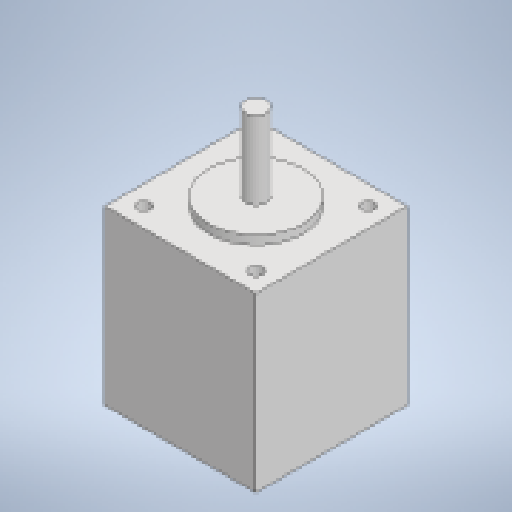
# Autodesk Inventor part: 35x40 stepper
Saved by Autodesk Inventor 2025 (Build 290162000, 162)
## iProperties
Created: 2025-09-03
Part Number: 35x40 stepper
Material: 一般
Document SubType Name: Modeling
Designer: gavin
Density: 1 g/cm^3
Appearance: 預設
Author: gavin
Autodesk Inventor part; units mm, degrees
ref_plane "YZ Plane" through (0, 0, 0) normal (1, 0, 0) x (0, 1, 0)
ref_plane "XZ Plane" through (0, 0, 0) normal (0, 1, 0) x (-1, 0, 0)
ref_plane "XY Plane" through (0, 0, 0) normal (0, 0, 1) x (1, 0, 0)
sketch "草圖1" plane through (0, 0, 0) normal (0, 1, 0) x (-1, 0, 0)
  line L0 (-17.5, 17.5) -> (17.5, 17.5)
  line L1 (17.5, 17.5) -> (17.5, -17.5)
  line L2 (17.5, -17.5) -> (-17.5, -17.5)
  line L3 (-17.5, -17.5) -> (-17.5, 17.5)
  line L4 (-17.5, 17.5) -> (17.5, -17.5) construction
  line L5 (17.5, 17.5) -> (-17.5, -17.5) construction
  point P0 (0, 0)
  dimension "d0" = 35
  dimension "d1" = 35
  constraints: 12 end point, 2 midpoint, 2 parallel, 1 horizontal, 1 perpendicular
  measures "d0" distance of L1.end L2.end
  measures "d1" distance of L0.end L1.end
extrude "擠出1" add sketch "草圖1" along normal blind 40
sketch "草圖2" plane through (0, 40, 0) normal (0, 1, 0) x (1, 0, 0)
  circle A0 centre (0, 0) radius 11
  dimension "d4" = 22
  constraints: 1 centre point, 1 coincident
  measures "d4" diameter of A0
extrude "擠出2" add sketch "草圖2" along normal blind 2
sketch "草圖3" plane through (0, 42, 0) normal (0, 1, 0) x (1, 0, 0)
  circle A0 centre (0, 0) radius 2.5
  dimension "d7" = 5
  constraints: 1 centre point, 1 coincident
  measures "d7" diameter of A0
extrude "擠出3" add sketch "草圖3" along normal blind 18
sketch "草圖4" plane through (0, 40, 0) normal (0, 1, 0) x (1, 0, 0)
  line L0 (13, -13) -> (-13, -13) construction
  line L1 (-13, -13) -> (-13, 13) construction
  line L2 (-13, 13) -> (13, 13) construction
  line L3 (13, 13) -> (13, -13) construction
  line L4 (13, -13) -> (-13, 13) construction
  line L5 (-13, -13) -> (13, 13) construction
  circle A0 centre (-13, -13) radius 1.5
  circle A1 centre (13, -13) radius 1.5
  circle A2 centre (13, 13) radius 1.5
  circle A3 centre (-13, 13) radius 1.5
  point P0 (0, 0)
  dimension "d10" = 26
  dimension "d11" = 26
  dimension "d12" = 3
  dimension "d15" = 360
  constraints: 12 end point, 4 centre point, 4 coincident, 2 midpoint, 2 parallel, 1 horizontal, 1 perpendicular, 13 other
  measures "d10" distance of L1.end L2.end
  measures "d11" distance of L0.end L1.end
  measures "d12" diameter of A0
extrude "擠出4" cut sketch "草圖4" against normal blind 2.5
